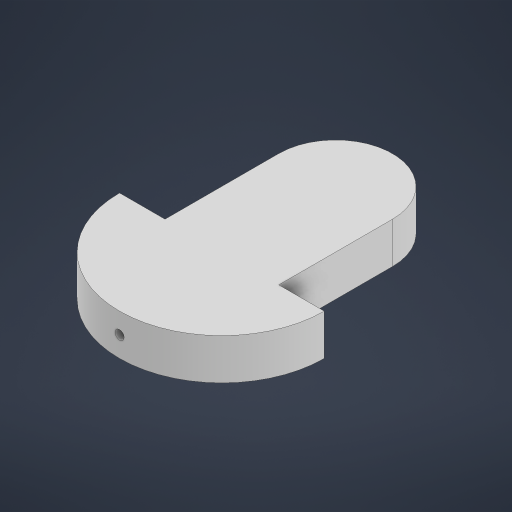
# Autodesk Inventor part: APM_001-1
Saved by Autodesk Inventor 2024 (Build 280153000, 153)
## iProperties
Created: 2023-05-12
Part Number: APM_001-1
Material: Genérico
Document SubType Name: Modeling
Designer: javie
Density: 1 g/cm^3
Appearance: Valor por defecto
Author: javie
Autodesk Inventor part; units mm, degrees
ref_plane "YZ Plane" through (0, 0, 0) normal (1, 0, 0) x (0, 1, 0)
ref_plane "XZ Plane" through (0, 0, 0) normal (0, 1, 0) x (-1, 0, 0)
sketch "Boceto1" plane through (0, 0, 0) normal (0, 1, 0) x (-1, 0, 0)
  arc A0 (-25, 25) -> (25, 25) centre (0, 25) ccw
  arc A1 (45, 75) -> (-45, 75) centre (0, 75) ccw
  line L0 (25, 25) -> (25, 75)
  line L1 (-25, 25) -> (-25, 75)
  line L2 (45, 75) -> (25, 75)
  line L3 (-25, 75) -> (-45, 75)
  point P0 (0, 0)
  dimension "d3" = 50
  dimension "d4" = 90
  constraints: 8 end point, 4 point on circle, 2 centre point, 2 perpendicular, 1 parallel
  measures "d3" diameter of A0
  measures "d4" diameter of A1
extrude "Extrusión1" add sketch "Boceto1" along normal blind 18
ref_plane "Plano de trabajo2" through (0, 0, 120) normal (0, 0, -1) x (-1, 0, 0)
sketch "Boceto3" plane through (0, 0, 120) normal (0, 0, -1) x (-1, 0, 0)
  circle A0 centre (0, 9) radius 2
  line L0 (45, 18) -> (-45, 18) projected
  point P0 (0, 0)
  dimension "d13" = 4
  dimension "d14" = 9
  constraints: 1 centre point
  measures "d13" diameter of A0
  measures "d14" distance from line of A0.centre L0
extrude "Extrusión3" add sketch "Boceto3" against normal blind 2
sketch "Boceto4" plane through (0, 9, 122) normal (0, 0, 1) x (1, 0, 0)
  circle A0 centre (0, 0) radius 2
  point P0 (0, -9)
  dimension "d17" = 4
  constraints: 1 centre point
  measures "d17" diameter of A0
extrude "Extrusión4" cut sketch "Boceto4" against normal blind 157.75
